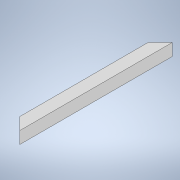
# Autodesk Inventor part: 5
Saved by Autodesk Inventor 2020.1 (Build 241239000, 239)
## iProperties
Created: 2019-12-19
Part Number: 5
Material: Generic
Document SubType Name: Modeling
Designer: super
Density: 1 g/cm^3
Appearance: Default
Author: super
Autodesk Inventor part; units mm, degrees
ref_plane "YZ Plane" through (0, 0, 0) normal (1, 0, 0) x (0, 1, 0)
ref_plane "XZ Plane" through (0, 0, 0) normal (0, 1, 0) x (-1, 0, 0)
ref_plane "XY Plane" through (0, 0, 0) normal (0, 0, 1) x (1, 0, 0)
sketch "Sketch1" plane through (0, 0, 0) normal (0, 1, 0) x (-1, 0, 0)
  line L0 (0, 0) -> (-6.35, 0)
  line L1 (-6.35, 0) -> (-6.35, -80)
  line L2 (-6.35, -80) -> (0, -80)
  line L3 (0, -80) -> (0, 0)
  dimension "d0" = 6.35
  dimension "d1" = 80
  constraints: 8 end point, 2 parallel, 1 horizontal, 1 perpendicular
  measures "d0" distance of L2.end L1.end
  measures "d1" distance of L1.end L0.end
extrude "Extrusion1" add sketch "Sketch1" along normal blind 6.35
sketch "Sketch2" plane through (0, 6.35, 0) normal (0, 1, 0) x (1, 0, 0)
  line L0 (0, 0) -> (6.35, 0) projected
  line L1 (6.35, 0) -> (0, 6.35)
  line L2 (0, 80) -> (0, 0) projected
  line L3 (6.35, 0) -> (15.3303, 0) construction
  line L4 (0, 6.35) -> (0, 0)
  line L5 (0, 0) -> (6.35, 0)
  dimension "d4" = 135
  constraints: 8 end point, 1 collinear, 1 equal length, 1 horizontal, 1 perpendicular, 1 point on line
  measures "d4" angle of L3 L1
extrude "Extrusion2" cut sketch "Sketch2" against normal blind 10
sketch "Sketch3" plane through (0, 6.35, 0) normal (0, 1, 0) x (1, 0, 0)
  line L0 (6.35, 80) -> (0, 73.65)
  line L1 (6.35, 80) -> (15.3303, 80) construction
  line L2 (0, 73.65) -> (0, 80)
  line L3 (6.35, 0) -> (6.35, 80) projected
  line L4 (6.35, 80) -> (0, 80) projected
  line L5 (0, 80) -> (6.35, 80)
  point P0 (0, 0)
  dimension "d7" = 135
  constraints: 8 end point, 1 equal length, 1 horizontal, 1 parallel, 1 perpendicular
  measures "d7" angle of L0 L1
extrude "Extrusion3" cut sketch "Sketch3" against normal blind 10
body "Solid1"
